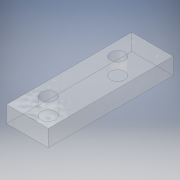
# Autodesk Inventor part: phone_holder_side_insert
Saved by Autodesk Inventor 2019 (Build 230136000, 136)
## iProperties
Created: 2019-02-17
Part Number: phone_holder_side_insert
Material: Acrylic, Clear
Document SubType Name: Modeling
Designer: suchanek
Density: 1.19 g/cm^3
Appearance: Transparent - Clear
Author: suchanek
Autodesk Inventor part; units mm, degrees
ref_plane "YZ Plane" through (0, 0, 0) normal (1, 0, 0) x (0, 1, 0)
ref_plane "XZ Plane" through (0, 0, 0) normal (0, 1, 0) x (-1, 0, 0)
ref_plane "XY Plane" through (0, 0, 0) normal (0, 0, 1) x (1, 0, 0)
sketch "Sketch2" plane through (0, 0, 0) normal (0, 1, 0) x (-1, 0, 0)
  line L0 (0, 0) -> (-15, 0)
  line L1 (-15, 0) -> (-15, 45)
  line L2 (-15, 45) -> (0, 45)
  line L3 (0, 45) -> (0, 0)
  circle A0 centre (-5, 10) radius 2.6
  circle A1 centre (-5, 35) radius 2.6
  dimension "d76" = 15
  dimension "d77" = 45
  dimension "d78" = 10
  dimension "d79" = 25
  dimension "d80" = 5
  dimension "d81" = 5.2
  constraints: 8 end point, 2 centre point, 2 parallel, 1 equal radius, 1 horizontal, 1 perpendicular, 1 vertical alignment
  measures "d76" distance of L1.end L2.end
  measures "d77" distance of L0.end L1.end
  measures "d78" distance from line of L0 A0.centre
  measures "d79" distance of A1.centre A0.centre
  measures "d80" distance from line of L3 A0.centre
  measures "d81" diameter of A1
extrude "Extrusion2" add sketch "Sketch2" along normal blind 6
body "Solid2"
